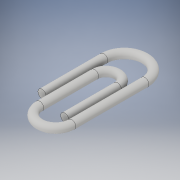
# Autodesk Inventor part: 練習一
Saved by Autodesk Inventor 2017 (Build 210142000, 142)
## iProperties
Part Number: 練習一
Material: 一般
Document SubType Name: Modeling
Designer: user
Density: 1 g/cm^3
Appearance: 預設
Author: user
Autodesk Inventor part; units mm, degrees
ref_plane "YZ Plane" through (0, 0, 0) normal (1, 0, 0) x (0, 1, 0)
ref_plane "XZ Plane" through (0, 0, 0) normal (0, 1, 0) x (-1, 0, 0)
sketch "草圖1" plane through (0, 0, 0) normal (0, 0, 1) x (1, 0, 0)
  line L0 (0, 0) -> (0, 6.75)
  arc A0 (4.5, 6.75) -> (0, 6.75) centre (2.25, 6.75) ccw
  line L1 (4.5, 6.75) -> (4.5, -1.25)
  arc A1 (1, -1.25) -> (4.5, -1.25) centre (2.75, -1.25) ccw
  line L2 (1, -1.25) -> (1, 4.75)
  arc A2 (3.5, 4.75) -> (1, 4.75) centre (2.25, 4.75) ccw
  line L3 (3.5, 4.75) -> (3.5, -1.0136)
  dimension "d0" = 3.5
  dimension "d2" = 4.5
  dimension "d3" = 2.5
  dimension "d4" = 8
  dimension "d5" = 4.75
  dimension "d6" = 6.75
  constraints: 8 end point, 6 point on circle, 6 tangent, 4 vertical, 3 centre point
  measures "d0" distance between parallel lines of L1 L2
  measures "d2" distance between parallel lines of L1 L0
  measures "d3" distance between parallel lines of L3 L2
  measures "d4" vertical distance of A1.centre A0.centre
  measures "d5" vertical distance of A2.centre L0.start
  measures "d6" vertical distance of A0.centre L0.start
ref_plane "工作平面1" through (0, 0, 0) normal (0, 1, 0) x (-1, 0, 0)
sketch "草圖2" plane through (0, 0, 0) normal (0, 1, 0) x (-1, 0, 0)
  circle A0 centre (0, 0) radius 0.45
  dimension "d7" = 0.9
  constraints: 1 centre point, 1 coincident
  measures "d7" diameter of A0
sweep "掃掠1" add profiles "草圖2" path "草圖1"
